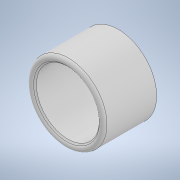
# Autodesk Inventor part: Github Test Part
Saved by Autodesk Inventor 2020 (Build 240168000, 168)
## iProperties
Created: 2021-02-03
Part Number: Github Test Part
Material: Generic
Document SubType Name: Modeling
Designer: sidsa
Density: 1 g/cm^3
Appearance: Default
Author: sidsa
Autodesk Inventor part; units mm, degrees
ref_plane "YZ Plane" through (0, 0, 0) normal (1, 0, 0) x (0, 1, 0)
ref_plane "XZ Plane" through (0, 0, 0) normal (0, 1, 0) x (-1, 0, 0)
ref_plane "XY Plane" through (0, 0, 0) normal (0, 0, 1) x (1, 0, 0)
sketch "Sketch1" plane through (0, 0, 0) normal (0, 0, 1) x (1, 0, 0)
  circle A0 centre (0, 0) radius 15.5308
  constraints: 1 centre point, 1 coincident
extrude "Extrusion1" add sketch "Sketch1" along normal blind 25.4
sketch "Sketch2" plane through (0, 0, 0) normal (0, 0, -1) x (-1, 0, 0)
  point P0 (0, 0)
sketch "Sketch3" plane through (0, 0, 25.4) normal (0, 0, 1) x (1, 0, 0)
  circle A0 centre (0, 0) radius 12.7
  dimension "d2" = 25.4
  constraints: 1 centre point, 1 coincident
  measures "d2" diameter of A0
extrude "Extrusion2" cut sketch "Sketch3" against normal blind 25.4
sketch "Sketch4" plane through (0, 0, 25.4) normal (0, 0, 1) x (1, 0, 0)
  circle A0 centre (0, 0) radius 13.97
  dimension "d5" = 27.94
  constraints: 1 centre point, 1 coincident
  measures "d5" diameter of A0
extrude "Extrusion3" cut sketch "Sketch4" against normal blind 5.08
fillet "Fillet1" radius 3.175 1 edges at (-13.97, 0, 20.32)
fillet "Fillet2" radius 3.175 1 edges at (-13.97, 0, 25.4)
fillet "Fillet3" radius 1.27 1 edges at (-15.5308, 0, 25.4)
body "Solid1"
